Autodesk Inventor part; units mm, degrees
(part 6 of 18)
  line L1143 (-10073.7191, -10027.8364) -> (-10073.719, -10027.8366)
  line L1144 (-10073.9178, -10027.8132) -> (-10073.9177, -10027.8133)
  line L1145 (-10073.9467, -10028.0617) -> (-10073.9468, -10028.0615)
  line L1146 (-10073.7727, -10026.5717) -> (-10073.7726, -10026.5718)
  line L1147 (-10073.6031, -10026.8432) -> (-10073.8017, -10026.82)
  line L1148 (-10073.8017, -10026.82) -> (-10073.7727, -10026.5717)
  line L1149 (-10073.603, -10026.8433) -> (-10073.6031, -10026.8432)
  line L1150 (-10075.4902, -10026.6227) -> (-10074.0004, -10026.7968)
  line L1151 (-10074.0004, -10026.7968) -> (-10074.1164, -10027.79)
  line L1152 (-10074.1164, -10027.79) -> (-10075.6063, -10027.6159)
  line L1153 (-10075.6063, -10027.6159) -> (-10075.4902, -10026.6227)
  line L1154 (-10074.1959, -10026.9515) -> (-10075.3355, -10026.8184)
  line L1155 (-10074.0004, -10026.7968) -> (-10074.1959, -10026.9515)
  line L1156 (-10075.4902, -10026.6227) -> (-10075.3355, -10026.8184)
  line L1157 (-10075.3355, -10026.8184) -> (-10075.4106, -10027.4614)
  line L1158 (-10075.6063, -10027.6159) -> (-10075.4106, -10027.4614)
  line L1159 (-10075.4106, -10027.4614) -> (-10074.271, -10027.5945)
  line L1160 (-10074.1164, -10027.79) -> (-10074.271, -10027.5945)
  line L1161 (-10074.271, -10027.5945) -> (-10074.1959, -10026.9515)
  circle A25 centre (-10075.0634, -10027.176) radius 0.1
  line L1162 (-10074.92, -10027.3438) -> (-10075.2416, -10027.3062)
  line L1163 (-10075.2416, -10027.3062) -> (-10075.2416, -10027.3062)
  line L1164 (-10074.92, -10027.3438) -> (-10075.2416, -10027.3062)
  line L1165 (-10074.92, -10027.3438) -> (-10074.92, -10027.3438)
  line L1166 (-10075.2416, -10027.3062) -> (-10075.2068, -10027.0083)
  line L1167 (-10075.2068, -10027.0083) -> (-10074.8852, -10027.0458)
  line L1168 (-10074.8852, -10027.0459) -> (-10074.8852, -10027.0458)
  line L1169 (-10074.8852, -10027.0458) -> (-10074.92, -10027.3438)
  line L1170 (-10074.8852, -10027.0459) -> (-10074.92, -10027.3438)
  line L1171 (-10065.1619, -10026.3344) -> (-10065.1851, -10026.5331)
  line L1172 (-10065.162, -10026.3343) -> (-10065.1619, -10026.3344)
  line L1173 (-10065.1852, -10026.5329) -> (-10065.162, -10026.3343)
  line L1174 (-10065.1851, -10026.5331) -> (-10065.1852, -10026.5329)
  line L1175 (-10064.9136, -10026.3635) -> (-10065.1619, -10026.3344)
  line L1176 (-10064.9137, -10026.3633) -> (-10064.9136, -10026.3635)
  line L1177 (-10065.162, -10026.3343) -> (-10064.9137, -10026.3633)
  line L1178 (-10066.1552, -10026.2184) -> (-10066.3836, -10026.1917)
  line L1179 (-10066.1784, -10026.4169) -> (-10066.1784, -10026.417)
  line L1180 (-10066.1552, -10026.2183) -> (-10066.1784, -10026.4169)
  line L1181 (-10066.4035, -10026.1892) -> (-10066.1552, -10026.2183)
  line L1182 (-10066.4035, -10026.1894) -> (-10066.4035, -10026.1892)
  line L1183 (-10065.1851, -10026.5331) -> (-10066.1784, -10026.417)
  line L1184 (-10064.6931, -10024.4763) -> (-10064.9136, -10026.3635)
  line L1185 (-10065.1852, -10026.5329) -> (-10066.1784, -10026.4169)
  line L1186 (-10066.4035, -10026.1892) -> (-10066.183, -10024.3021)
  line L1187 (-10064.6932, -10024.4761) -> (-10064.9137, -10026.3633)
  line L1188 (-10065.9115, -10024.1324) -> (-10064.9183, -10024.2485)
  line L1189 (-10064.9182, -10024.2486) -> (-10064.9414, -10024.4471)
  line L1190 (-10064.6932, -10024.4761) -> (-10064.9415, -10024.4471)
  line L1191 (-10064.9415, -10024.4471) -> (-10064.9183, -10024.2485)
  line L1192 (-10064.9183, -10024.2485) -> (-10064.9182, -10024.2486)
  line L1193 (-10064.6931, -10024.4763) -> (-10064.6932, -10024.4761)
  line L1194 (-10065.9115, -10024.1324) -> (-10065.9347, -10024.3311)
  line L1195 (-10065.9347, -10024.3311) -> (-10066.183, -10024.3021)
  line L1196 (-10066.132, -10026.0196) -> (-10065.9579, -10024.5297)
  line L1197 (-10065.9579, -10024.5297) -> (-10064.9647, -10024.6458)
  line L1198 (-10064.9647, -10024.6458) -> (-10065.1388, -10026.1357)
  line L1199 (-10065.1388, -10026.1357) -> (-10066.132, -10026.0196)
  line L1200 (-10065.8032, -10024.7254) -> (-10065.9364, -10025.865)
  line L1201 (-10065.9579, -10024.5297) -> (-10065.8032, -10024.7254)
  line L1202 (-10066.132, -10026.0196) -> (-10065.9364, -10025.865)
  line L1203 (-10065.9364, -10025.865) -> (-10065.2934, -10025.9402)
  line L1204 (-10065.1388, -10026.1357) -> (-10065.2934, -10025.9402)
  line L1205 (-10065.2934, -10025.9402) -> (-10065.1602, -10024.8006)
  line L1206 (-10064.9647, -10024.6458) -> (-10065.1602, -10024.8006)
  line L1207 (-10065.1602, -10024.8006) -> (-10065.8032, -10024.7254)
  circle A26 centre (-10065.5787, -10025.5929) radius 0.1
  line L1208 (-10065.4109, -10025.4495) -> (-10065.4485, -10025.7711)
  line L1209 (-10065.4485, -10025.7712) -> (-10065.4485, -10025.7711)
  line L1210 (-10065.4109, -10025.4495) -> (-10065.4485, -10025.7712)
  line L1211 (-10065.4109, -10025.4495) -> (-10065.4109, -10025.4495)
  line L1212 (-10065.4485, -10025.7711) -> (-10065.7465, -10025.7363)
  line L1213 (-10065.7465, -10025.7363) -> (-10065.7465, -10025.7363)
  line L1214 (-10065.4485, -10025.7712) -> (-10065.7465, -10025.7363)
  line L1215 (-10065.7465, -10025.7363) -> (-10065.7089, -10025.4147)
  line L1216 (-10065.7089, -10025.4147) -> (-10065.4109, -10025.4495)
  line L1217 (-10077.2652, -10022.532) -> (-10077.0665, -10022.532)
  line L1218 (-10077.0665, -10022.532) -> (-10077.0665, -10022.782)
  line L1219 (-10077.0665, -10021.532) -> (-10077.2652, -10021.532)
  line L1220 (-10077.0665, -10021.282) -> (-10077.0665, -10021.532)
  line L1221 (-10075.017, -10021.282) -> (-10075.017, -10021.532)
  line L1222 (-10075.1793, -10021.282) -> (-10075.017, -10021.282)
  line L1223 (-10074.9807, -10021.532) -> (-10075.1793, -10021.532)
  line L1224 (-10075.1793, -10021.532) -> (-10075.1793, -10021.282)
  line L1225 (-10074.8184, -10021.532) -> (-10074.9807, -10021.532)
  line L1226 (-10074.8184, -10021.532) -> (-10074.8184, -10022.532)
  line L1227 (-10077.2652, -10022.532) -> (-10077.2652, -10021.532)
  line L1228 (-10077.0665, -10021.282) -> (-10075.1793, -10021.282)
  line L1229 (-10075.1793, -10022.782) -> (-10077.0665, -10022.782)
  line L1230 (-10074.9807, -10021.532) -> (-10074.9807, -10022.532)
  line L1231 (-10075.017, -10022.532) -> (-10075.017, -10022.782)
  line L1232 (-10075.1793, -10022.782) -> (-10075.1793, -10022.532)
  line L1233 (-10075.1793, -10022.532) -> (-10074.9807, -10022.532)
  line L1234 (-10074.9807, -10022.532) -> (-10074.8184, -10022.532)
  line L1235 (-10075.017, -10022.782) -> (-10075.1793, -10022.782)
  line L1236 (-10076.8679, -10021.532) -> (-10075.378, -10021.532)
  line L1237 (-10075.378, -10021.532) -> (-10075.378, -10022.532)
  line L1238 (-10075.378, -10022.532) -> (-10076.8679, -10022.532)
  line L1239 (-10076.8679, -10022.532) -> (-10076.8679, -10021.532)
  line L1240 (-10075.4372, -10021.7083) -> (-10076.5768, -10021.7083)
  line L1241 (-10075.378, -10021.532) -> (-10075.4372, -10021.7083)
  line L1242 (-10076.8679, -10021.532) -> (-10076.5768, -10021.7083)
  line L1243 (-10076.5768, -10021.7083) -> (-10076.5768, -10022.3557)
  line L1244 (-10076.8679, -10022.532) -> (-10076.5768, -10022.3557)
  line L1245 (-10076.5768, -10022.3557) -> (-10075.4372, -10022.3557)
  line L1246 (-10075.378, -10022.532) -> (-10075.4372, -10022.3557)
  line L1247 (-10075.4372, -10022.3557) -> (-10075.4372, -10021.7083)
  ellipse E653 centre (-10076.2961, -10022.032) end of major axis (-10076.2961, -10021.932) minor radius 0.0993
  ellipse E654 centre (-10076.2903, -10022.032) end of major axis (-10076.2903, -10021.932) minor radius 0.0993 (-10076.2903, -10022.132) -> (-10076.2903, -10021.932) ccw
  line L1248 (-10076.2903, -10022.132) -> (-10076.2961, -10022.132)
  line L1249 (-10076.2903, -10021.932) -> (-10076.2961, -10021.932)
  line L1250 (-10076.1295, -10022.182) -> (-10076.4512, -10022.182)
  line L1251 (-10076.1063, -10022.182) -> (-10076.1295, -10022.182)
  line L1252 (-10076.4512, -10022.182) -> (-10076.4512, -10021.882)
  line L1253 (-10076.4512, -10021.882) -> (-10076.1295, -10021.882)
  line L1254 (-10076.1063, -10021.882) -> (-10076.1295, -10021.882)
  line L1255 (-10076.1295, -10021.882) -> (-10076.1295, -10022.182)
  line L1256 (-10076.1063, -10021.882) -> (-10076.1063, -10022.182)
  line L1257 (-10066.5495, -10020.047) -> (-10066.5495, -10020.247)
  line L1258 (-10066.7118, -10020.247) -> (-10066.7118, -10020.047)
  line L1259 (-10066.5495, -10020.247) -> (-10066.7118, -10020.247)
  line L1260 (-10066.4635, -10020.047) -> (-10066.3012, -10020.047)
  line L1261 (-10066.7118, -10020.047) -> (-10066.4635, -10020.047)
  line L1262 (-10067.7051, -10020.047) -> (-10067.7051, -10020.247)
  line L1263 (-10067.9534, -10020.047) -> (-10067.7051, -10020.047)
  line L1264 (-10066.5495, -10017.947) -> (-10066.5495, -10018.147)
  line L1265 (-10066.4635, -10018.147) -> (-10066.7118, -10018.147)
  line L1266 (-10066.7118, -10018.147) -> (-10066.7118, -10017.947)
  line L1267 (-10066.7118, -10017.947) -> (-10066.5495, -10017.947)
  line L1268 (-10066.3012, -10018.147) -> (-10066.4635, -10018.147)
  line L1269 (-10066.3012, -10018.147) -> (-10066.3012, -10020.047)
  line L1270 (-10066.7118, -10020.247) -> (-10067.7051, -10020.247)
  line L1271 (-10067.9534, -10020.047) -> (-10067.9534, -10018.147)
  line L1272 (-10066.4635, -10018.147) -> (-10066.4635, -10020.047)
  line L1273 (-10067.7051, -10017.947) -> (-10066.7118, -10017.947)
  line L1274 (-10067.7051, -10017.947) -> (-10067.7051, -10018.147)
  line L1275 (-10067.7051, -10018.147) -> (-10067.9534, -10018.147)
  line L1276 (-10067.7051, -10019.847) -> (-10067.7051, -10018.347)
  line L1277 (-10067.7051, -10018.347) -> (-10066.7118, -10018.347)
  line L1278 (-10066.7118, -10018.347) -> (-10066.7118, -10019.847)
  line L1279 (-10066.7118, -10019.847) -> (-10067.7051, -10019.847)
  line L1280 (-10067.414, -10018.5233) -> (-10067.414, -10019.6707)
  line L1281 (-10067.7051, -10018.347) -> (-10067.414, -10018.5233)
  line L1282 (-10067.7051, -10019.847) -> (-10067.414, -10019.6707)
  line L1283 (-10067.414, -10019.6707) -> (-10066.771, -10019.6707)
  line L1284 (-10066.7118, -10019.847) -> (-10066.771, -10019.6707)
  line L1285 (-10066.771, -10019.6707) -> (-10066.771, -10018.5233)
  line L1286 (-10066.7118, -10018.347) -> (-10066.771, -10018.5233)
  line L1287 (-10066.771, -10018.5233) -> (-10067.414, -10018.5233)
  ellipse E655 centre (-10067.1215, -10019.3589) end of major axis (-10067.1215, -10019.2589) minor radius 0.0993
  ellipse E656 centre (-10067.1157, -10019.3589) end of major axis (-10067.1157, -10019.2589) minor radius 0.0993 (-10067.1157, -10019.4589) -> (-10067.1157, -10019.2589) ccw
  line L1288 (-10067.1157, -10019.4589) -> (-10067.1215, -10019.4589)
  line L1289 (-10067.1157, -10019.2589) -> (-10067.1215, -10019.2589)
  line L1290 (-10066.9667, -10019.197) -> (-10066.9667, -10019.5208)
  line L1291 (-10066.9435, -10019.5208) -> (-10066.9667, -10019.5208)
  line L1292 (-10066.9435, -10019.197) -> (-10066.9435, -10019.5208)
  line L1293 (-10066.9435, -10019.197) -> (-10066.9667, -10019.197)
  line L1294 (-10066.9667, -10019.5208) -> (-10067.2647, -10019.5208)
  line L1295 (-10067.2647, -10019.5208) -> (-10067.2647, -10019.197)
  line L1296 (-10067.2647, -10019.197) -> (-10066.9667, -10019.197)
  line L1297 (-10064.9414, -10013.7468) -> (-10064.9182, -10013.9454)
  line L1298 (-10064.9183, -10013.9455) -> (-10064.9415, -10013.7468)
  line L1299 (-10064.9182, -10013.9454) -> (-10064.9183, -10013.9455)
  line L1300 (-10064.6932, -10013.7178) -> (-10064.6931, -10013.7177)
  line L1301 (-10064.9415, -10013.7468) -> (-10064.6932, -10013.7178)
  line L1302 (-10065.9347, -10013.8629) -> (-10065.9115, -10014.0615)
  line L1303 (-10066.183, -10013.8919) -> (-10065.9347, -10013.8629)
  line L1304 (-10066.3836, -10012.0023) -> (-10066.1552, -10011.9756)
  line L1305 (-10066.4035, -10012.0047) -> (-10066.4035, -10012.0046)
  line L1306 (-10066.1784, -10011.7771) -> (-10066.1552, -10011.9757)
  line L1307 (-10066.1552, -10011.9757) -> (-10066.4035, -10012.0047)
  line L1308 (-10066.1784, -10011.7769) -> (-10066.1784, -10011.7771)
  line L1309 (-10066.1784, -10011.7769) -> (-10065.1851, -10011.6609)
  line L1310 (-10064.9136, -10011.8305) -> (-10064.6931, -10013.7177)
  line L1311 (-10064.9183, -10013.9455) -> (-10065.9115, -10014.0615)
  line L1312 (-10066.183, -10013.8919) -> (-10066.4035, -10012.0047)
  line L1313 (-10064.9137, -10011.8307) -> (-10064.6932, -10013.7178)
  line L1314 (-10066.1784, -10011.7771) -> (-10065.1852, -10011.661)
  line L1315 (-10065.1851, -10011.6609) -> (-10065.1619, -10011.8595)
  line L1316 (-10065.1619, -10011.8595) -> (-10064.9136, -10011.8305)
  line L1317 (-10064.9137, -10011.8307) -> (-10065.162, -10011.8597)
  line L1318 (-10065.162, -10011.8597) -> (-10065.1852, -10011.661)
  line L1319 (-10065.1852, -10011.661) -> (-10065.1851, -10011.6609)
  line L1320 (-10065.162, -10011.8597) -> (-10065.1619, -10011.8595)
  line L1321 (-10064.9136, -10011.8305) -> (-10064.9137, -10011.8307)
  line L1322 (-10065.9579, -10013.6642) -> (-10066.132, -10012.1744)
  line L1323 (-10066.132, -10012.1744) -> (-10065.1388, -10012.0583)
  line L1324 (-10065.1388, -10012.0583) -> (-10064.9647, -10013.5482)
  line L1325 (-10064.9647, -10013.5482) -> (-10065.9579, -10013.6642)
  line L1326 (-10065.9364, -10012.329) -> (-10065.8032, -10013.4685)
  line L1327 (-10066.132, -10012.1744) -> (-10065.9364, -10012.329)
  line L1328 (-10065.9579, -10013.6642) -> (-10065.8032, -10013.4685)
  line L1329 (-10065.8032, -10013.4685) -> (-10065.1602, -10013.3934)
  line L1330 (-10064.9647, -10013.5482) -> (-10065.1602, -10013.3934)
  line L1331 (-10065.1602, -10013.3934) -> (-10065.2934, -10012.2538)
  line L1332 (-10065.1388, -10012.0583) -> (-10065.2934, -10012.2538)
  line L1333 (-10065.2934, -10012.2538) -> (-10065.9364, -10012.329)
  circle A27 centre (-10065.5179, -10013.1214) radius 0.1
  line L1334 (-10065.3877, -10012.9431) -> (-10065.3501, -10013.2648)
  line L1335 (-10065.3501, -10013.2647) -> (-10065.3501, -10013.2648)
  line L1336 (-10065.3877, -10012.9431) -> (-10065.3501, -10013.2647)
  line L1337 (-10065.3877, -10012.9431) -> (-10065.3877, -10012.9431)
  line L1338 (-10065.3501, -10013.2648) -> (-10065.6481, -10013.2996)
  line L1339 (-10065.6481, -10013.2996) -> (-10065.6857, -10012.9779)
  line L1340 (-10065.6857, -10012.9779) -> (-10065.6857, -10012.9779)
  line L1341 (-10065.6857, -10012.9779) -> (-10065.3877, -10012.9431)
  line L1342 (-10065.6857, -10012.9779) -> (-10065.3877, -10012.9431)
  line L1343 (-10079.6036, -10026.2937) -> (-10079.8027, -10026.2748)
  line L1344 (-10079.8027, -10026.2747) -> (-10079.6036, -10026.2936)
  line L1345 (-10079.8027, -10026.2748) -> (-10079.8027, -10026.2747)
  line L1346 (-10079.6272, -10026.5425) -> (-10079.6272, -10026.5426)
  line L1347 (-10079.6036, -10026.2936) -> (-10079.6272, -10026.5425)
  line L1348 (-10079.5092, -10025.298) -> (-10079.7083, -10025.2792)
  line L1349 (-10079.4856, -10025.0492) -> (-10079.5092, -10025.298)
  line L1350 (-10079.407, -10026.5634) -> (-10079.6272, -10026.5426)
  line L1351 (-10079.8027, -10026.2747) -> (-10079.7083, -10025.2792)
  line L1352 (-10079.4856, -10025.0492) -> (-10077.5941, -10025.2284)
  line L1353 (-10077.8748, -10026.7086) -> (-10079.6272, -10026.5425)
  line L1354 (-10077.4186, -10025.4962) -> (-10077.433, -10025.6486)
  line L1355 (-10077.5941, -10025.2284) -> (-10077.5941, -10025.2285)
  line L1356 (-10077.4186, -10025.4962) -> (-10077.6177, -10025.4773)
  line L1357 (-10077.6177, -10025.4773) -> (-10077.5941, -10025.2284)
  line L1358 (-10077.4186, -10025.4963) -> (-10077.4186, -10025.4962)
  line L1359 (-10079.3101, -10025.3169) -> (-10077.8168, -10025.4585)
  line L1360 (-10077.8168, -10025.4585) -> (-10077.9112, -10026.454)
  line L1361 (-10077.9112, -10026.454) -> (-10079.4045, -10026.3125)
  line L1362 (-10079.4045, -10026.3125) -> (-10079.3101, -10025.3169)
  line L1363 (-10078.009, -10025.6174) -> (-10079.1512, -10025.5092)
  line L1364 (-10077.8168, -10025.4585) -> (-10078.009, -10025.6174)
  line L1365 (-10079.3101, -10025.3169) -> (-10079.1512, -10025.5092)
  line L1366 (-10079.1512, -10025.5092) -> (-10079.2123, -10026.1536)
  line L1367 (-10079.4045, -10026.3125) -> (-10079.2123, -10026.1536)
  line L1368 (-10079.2123, -10026.1536) -> (-10078.0701, -10026.2619)
  line L1369 (-10077.9112, -10026.454) -> (-10078.0701, -10026.2619)
  line L1370 (-10078.0701, -10026.2619) -> (-10078.009, -10025.6174)
  circle A28 centre (-10078.8714, -10025.8608) radius 0.1
  line L1371 (-10078.7243, -10026.0254) -> (-10079.0467, -10025.9949)
  line L1372 (-10078.7243, -10026.0254) -> (-10079.0467, -10025.9949)
  line L1373 (-10079.0467, -10025.9949) -> (-10079.0184, -10025.6962)
  line L1374 (-10079.0184, -10025.6962) -> (-10078.696, -10025.7267)
  line L1375 (-10078.696, -10025.7267) -> (-10078.7243, -10026.0254)
  line L1376 (-10068.9906, -10024.8034) -> (-10068.9906, -10024.8035)
  line L1377 (-10069.0095, -10025.0025) -> (-10068.9906, -10024.8034)
  line L1378 (-10069.0095, -10025.0026) -> (-10069.0095, -10025.0025)
  line L1379 (-10068.7417, -10024.827) -> (-10068.7417, -10024.8271)
  line L1380 (-10068.9906, -10024.8034) -> (-10068.7417, -10024.827)
  line L1381 (-10070.005, -10024.9081) -> (-10070.005, -10024.9082)
  line L1382 (-10069.9861, -10024.709) -> (-10070.005, -10024.9081)
  line L1383 (-10070.235, -10024.6854) -> (-10069.9861, -10024.709)
  line L1384 (-10070.235, -10024.6856) -> (-10070.235, -10024.6854)
  line L1385 (-10069.0095, -10025.0025) -> (-10070.005, -10024.9081)
  line L1386 (-10070.235, -10024.6854) -> (-10070.0557, -10022.7939)
  line L1387 (-10068.5624, -10022.9355) -> (-10068.7417, -10024.827)
  line L1388 (-10069.788, -10022.6184) -> (-10068.7924, -10022.7128)
  line L1389 (-10068.5624, -10022.9355) -> (-10068.8113, -10022.9119)
  line L1390 (-10068.8113, -10022.9119) -> (-10068.7924, -10022.7128)
  line L1391 (-10068.7924, -10022.7128) -> (-10068.7924, -10022.7129)
  line L1392 (-10068.5624, -10022.9356) -> (-10068.5624, -10022.9355)
  line L1393 (-10069.788, -10022.6184) -> (-10069.8069, -10022.8175)
  line L1394 (-10069.8069, -10022.8175) -> (-10070.0557, -10022.7939)
  line L1395 (-10069.9673, -10024.5099) -> (-10069.8257, -10023.0166)
  line L1396 (-10069.8257, -10023.0166) -> (-10068.8302, -10023.111)
  line L1397 (-10068.8302, -10023.111) -> (-10068.9717, -10024.6043)
  line L1398 (-10068.9717, -10024.6043) -> (-10069.9673, -10024.5099)
  line L1399 (-10069.6668, -10023.2089) -> (-10069.7751, -10024.3511)
  line L1400 (-10069.8257, -10023.0166) -> (-10069.6668, -10023.2089)
  line L1401 (-10069.9673, -10024.5099) -> (-10069.7751, -10024.3511)
  line L1402 (-10069.7751, -10024.3511) -> (-10069.1306, -10024.4122)
  line L1403 (-10068.9717, -10024.6043) -> (-10069.1306, -10024.4122)
  line L1404 (-10069.1306, -10024.4122) -> (-10069.0224, -10023.27)
  line L1405 (-10068.8302, -10023.111) -> (-10069.0224, -10023.27)
  line L1406 (-10069.0224, -10023.27) -> (-10069.6668, -10023.2089)
  circle A29 centre (-10069.4234, -10024.0713) radius 0.1
  line L1407 (-10069.2588, -10023.9242) -> (-10069.2894, -10024.2466)
  line L1408 (-10069.2894, -10024.2466) -> (-10069.5881, -10024.2183)
  line L1409 (-10069.2894, -10024.2466) -> (-10069.5881, -10024.2183)
  line L1410 (-10069.5881, -10024.2183) -> (-10069.5575, -10023.8959)
  line L1411 (-10069.5575, -10023.8959) -> (-10069.2588, -10023.9242)
  line L1412 (-10080.8297, -10022.532) -> (-10080.6306, -10022.532)
  line L1413 (-10080.6306, -10022.532) -> (-10080.6306, -10022.782)
  line L1414 (-10080.6306, -10021.532) -> (-10080.8297, -10021.532)
  line L1415 (-10080.6306, -10021.282) -> (-10080.6306, -10021.532)
  line L1416 (-10080.8297, -10022.532) -> (-10080.8297, -10021.532)
  line L1417 (-10080.6306, -10021.282) -> (-10078.8245, -10021.282)
  line L1418 (-10078.8245, -10022.782) -> (-10080.6306, -10022.782)
  line L1419 (-10080.4314, -10021.532) -> (-10079.0234, -10021.532)
  line L1420 (-10079.0234, -10022.532) -> (-10080.4314, -10022.532)
  line L1421 (-10080.4314, -10022.532) -> (-10080.4314, -10021.532)
  line L1422 (-10079.6809, -10021.7083) -> (-10080.1616, -10021.7083)
  line L1423 (-10080.4314, -10021.532) -> (-10080.1616, -10021.7083)
  line L1424 (-10080.1616, -10021.7083) -> (-10080.1616, -10022.3557)
  line L1425 (-10080.4314, -10022.532) -> (-10080.1616, -10022.3557)
  line L1426 (-10080.1616, -10022.3557) -> (-10079.6809, -10022.3557)
  ellipse E657 centre (-10079.8748, -10022.032) end of major axis (-10079.8748, -10021.932) minor radius 0.0996
  ellipse E658 centre (-10079.8701, -10022.032) end of major axis (-10079.8701, -10021.932) minor radius 0.0996 (-10079.8701, -10022.132) -> (-10079.8701, -10021.932) ccw
  line L1427 (-10079.8701, -10022.132) -> (-10079.8748, -10022.132)
  line L1428 (-10079.8701, -10021.932) -> (-10079.8748, -10021.932)
  line L1429 (-10079.7089, -10022.182) -> (-10080.0313, -10022.182)
  line L1430 (-10079.69, -10022.182) -> (-10079.7089, -10022.182)
  line L1431 (-10080.0313, -10022.182) -> (-10080.0313, -10021.882)
  line L1432 (-10080.0313, -10021.882) -> (-10079.7089, -10021.882)
  line L1433 (-10079.69, -10021.882) -> (-10079.7089, -10021.882)
  line L1434 (-10079.7089, -10021.882) -> (-10079.7089, -10022.182)
  line L1435 (-10079.69, -10021.882) -> (-10079.69, -10022.182)
  line L1436 (-10070.252, -10020.247) -> (-10070.252, -10020.047)
  line L1437 (-10070.2216, -10020.247) -> (-10070.252, -10020.247)
  line L1438 (-10070.0031, -10020.047) -> (-10069.9732, -10020.047)
  line L1439 (-10070.252, -10020.047) -> (-10070.0031, -10020.047)
  line L1440 (-10071.2476, -10020.047) -> (-10071.2476, -10020.247)
  line L1441 (-10071.4965, -10020.047) -> (-10071.2476, -10020.047)
  line L1442 (-10070.252, -10020.247) -> (-10071.2476, -10020.247)
  line L1443 (-10071.4965, -10020.047) -> (-10071.4965, -10018.147)
  line L1444 (-10070.0031, -10018.147) -> (-10070.0031, -10020.047)
  line L1445 (-10071.2476, -10017.947) -> (-10070.252, -10017.947)
  line L1446 (-10070.0031, -10018.147) -> (-10070.252, -10018.147)
  line L1447 (-10070.252, -10018.147) -> (-10070.252, -10017.947)
  line L1448 (-10070.252, -10017.947) -> (-10070.2216, -10017.947)
  line L1449 (-10069.9732, -10018.147) -> (-10070.0031, -10018.147)
  line L1450 (-10071.2476, -10017.947) -> (-10071.2476, -10018.147)
  line L1451 (-10071.2476, -10018.147) -> (-10071.4965, -10018.147)
  line L1452 (-10071.2476, -10019.847) -> (-10071.2476, -10018.347)
  line L1453 (-10071.2476, -10018.347) -> (-10070.252, -10018.347)
  line L1454 (-10070.252, -10018.347) -> (-10070.252, -10019.847)
  line L1455 (-10070.252, -10019.847) -> (-10071.2476, -10019.847)
  line L1456 (-10071.2476, -10018.347) -> (-10071.1549, -10018.4076)
  line L1457 (-10071.2476, -10019.847) -> (-10071.1549, -10019.7864)
  line L1458 (-10070.252, -10019.847) -> (-10070.2784, -10019.7898)
  line L1459 (-10070.252, -10018.347) -> (-10070.2784, -10018.4042)
  line L1460 (-10068.7924, -10015.4812) -> (-10068.8113, -10015.2821)
  line L1461 (-10068.7924, -10015.4811) -> (-10068.7924, -10015.4812)
  line L1462 (-10068.5624, -10015.2585) -> (-10068.5624, -10015.2584)
  line L1463 (-10068.8113, -10015.2821) -> (-10068.5624, -10015.2585)
  line L1464 (-10069.8069, -10015.3765) -> (-10069.788, -10015.5756)
  line L1465 (-10070.0557, -10015.4001) -> (-10069.8069, -10015.3765)
  line L1466 (-10068.7924, -10015.4812) -> (-10069.788, -10015.5756)
  line L1467 (-10070.0557, -10015.4001) -> (-10070.235, -10013.5085)
  line L1468 (-10068.7417, -10013.367) -> (-10068.5624, -10015.2585)
  line L1469 (-10070.005, -10013.2858) -> (-10069.0095, -10013.1915)
  line L1470 (-10070.235, -10013.5085) -> (-10070.235, -10013.5084)
  line L1471 (-10070.005, -10013.2858) -> (-10069.9861, -10013.4849)
  line L1472 (-10069.9861, -10013.4849) -> (-10070.235, -10013.5085)
  line L1473 (-10070.005, -10013.2857) -> (-10070.005, -10013.2858)
  line L1474 (-10068.7417, -10013.367) -> (-10068.9906, -10013.3906)
  line L1475 (-10068.9906, -10013.3906) -> (-10069.0095, -10013.1915)
  line L1476 (-10069.0095, -10013.1915) -> (-10069.0095, -10013.1914)
  line L1477 (-10068.9906, -10013.3906) -> (-10068.9906, -10013.3905)
  line L1478 (-10068.7417, -10013.3669) -> (-10068.7417, -10013.367)
  line L1479 (-10069.8257, -10015.1774) -> (-10069.9673, -10013.684)
  line L1480 (-10069.9673, -10013.684) -> (-10068.9717, -10013.5897)
  line L1481 (-10068.9717, -10013.5897) -> (-10068.8302, -10015.083)
  line L1482 (-10068.8302, -10015.083) -> (-10069.8257, -10015.1774)
  line L1483 (-10069.7751, -10013.8429) -> (-10069.6668, -10014.9851)
  line L1484 (-10069.9673, -10013.684) -> (-10069.7751, -10013.8429)
  line L1485 (-10069.8257, -10015.1774) -> (-10069.6668, -10014.9851)
  line L1486 (-10069.6668, -10014.9851) -> (-10069.0224, -10014.924)
  line L1487 (-10068.8302, -10015.083) -> (-10069.0224, -10014.924)
  line L1488 (-10069.0224, -10014.924) -> (-10069.1306, -10013.7818)
  line L1489 (-10068.9717, -10013.5897) -> (-10069.1306, -10013.7818)
  line L1490 (-10069.1306, -10013.7818) -> (-10069.7751, -10013.8429)
  circle A30 centre (-10069.374, -10014.6442) radius 0.1
  line L1491 (-10069.24, -10014.4689) -> (-10069.2094, -10014.7912)
  line L1492 (-10069.2094, -10014.7912) -> (-10069.5081, -10014.8195)
  line L1493 (-10069.5081, -10014.8195) -> (-10069.5386, -10014.4972)
  line L1494 (-10069.5386, -10014.4972) -> (-10069.24, -10014.4689)
  line L1495 (-10069.5386, -10014.4972) -> (-10069.24, -10014.4688)
  line L1496 (-10051.002, -10021.597) -> (-10051.202, -10021.597)
  line L1497 (-10051.202, -10021.597) -> (-10051.202, -10021.347)
  line L1498 (-10051.202, -10022.597) -> (-10051.002, -10022.597)
  line L1499 (-10051.202, -10022.847) -> (-10051.202, -10022.597)
  line L1500 (-10051.002, -10021.597) -> (-10051.002, -10022.597)
  line L1501 (-10051.202, -10022.847) -> (-10053.102, -10022.847)
  line L1502 (-10053.102, -10021.347) -> (-10051.202, -10021.347)
  line L1503 (-10053.302, -10022.597) -> (-10053.302, -10021.597)
  line L1504 (-10053.102, -10021.347) -> (-10053.102, -10021.597)
  line L1505 (-10053.102, -10021.597) -> (-10053.302, -10021.597)
  line L1506 (-10053.302, -10022.597) -> (-10053.102, -10022.597)
  line L1507 (-10053.102, -10022.597) -> (-10053.102, -10022.847)
  line L1508 (-10051.402, -10022.597) -> (-10052.902, -10022.597)
  line L1509 (-10052.902, -10022.597) -> (-10052.902, -10021.597)
  line L1510 (-10052.902, -10021.597) -> (-10051.402, -10021.597)
  line L1511 (-10051.402, -10021.597) -> (-10051.402, -10022.597)
  line L1512 (-10052.7257, -10022.4207) -> (-10051.5783, -10022.4207)
  line L1513 (-10052.902, -10022.597) -> (-10052.7257, -10022.4207)
  line L1514 (-10051.402, -10022.597) -> (-10051.5783, -10022.4207)
  line L1515 (-10051.5783, -10022.4207) -> (-10051.5783, -10021.7733)
  line L1516 (-10051.402, -10021.597) -> (-10051.5783, -10021.7733)
  line L1517 (-10051.5783, -10021.7733) -> (-10052.7257, -10021.7733)
  line L1518 (-10052.902, -10021.597) -> (-10052.7257, -10021.7733)
  line L1519 (-10052.7257, -10021.7733) -> (-10052.7257, -10022.4207)
  circle A31 centre (-10051.8901, -10022.097) radius 0.1
  line L1520 (-10052.052, -10021.947) -> (-10051.7282, -10021.947)
  line L1521 (-10051.7282, -10021.947) -> (-10051.7282, -10022.247)
  line L1522 (-10051.7282, -10022.247) -> (-10052.052, -10022.247)
  line L1523 (-10052.052, -10022.247) -> (-10052.052, -10021.947)
  line L1524 (-10061.6, -10017.947) -> (-10061.6, -10018.147)
  line L1525 (-10061.6, -10018.147) -> (-10061.85, -10018.147)
  line L1526 (-10060.6, -10018.147) -> (-10060.6, -10017.947)
  line L1527 (-10060.35, -10018.147) -> (-10060.6, -10018.147)
  line L1528 (-10061.6, -10017.947) -> (-10060.6, -10017.947)
  line L1529 (-10060.35, -10018.147) -> (-10060.35, -10020.047)
  line L1530 (-10061.85, -10020.047) -> (-10061.85, -10018.147)
  line L1531 (-10060.6, -10020.247) -> (-10061.6, -10020.247)
  line L1532 (-10061.85, -10020.047) -> (-10061.6, -10020.047)
  line L1533 (-10061.6, -10020.047) -> (-10061.6, -10020.247)
  line L1534 (-10060.6, -10020.247) -> (-10060.6, -10020.047)
  line L1535 (-10060.6, -10020.047) -> (-10060.35, -10020.047)
  line L1536 (-10060.6, -10018.347) -> (-10060.6, -10019.847)
  line L1537 (-10060.6, -10019.847) -> (-10061.6, -10019.847)
  line L1538 (-10061.6, -10019.847) -> (-10061.6, -10018.347)
  line L1539 (-10061.6, -10018.347) -> (-10060.6, -10018.347)
  line L1540 (-10060.7763, -10019.6707) -> (-10060.7763, -10018.5233)
  line L1541 (-10060.6, -10019.847) -> (-10060.7763, -10019.6707)
  line L1542 (-10060.6, -10018.347) -> (-10060.7763, -10018.5233)
  line L1543 (-10060.7763, -10018.5233) -> (-10061.4237, -10018.5233)
  line L1544 (-10061.6, -10018.347) -> (-10061.4237, -10018.5233)
  line L1545 (-10061.4237, -10018.5233) -> (-10061.4237, -10019.6707)
  line L1546 (-10061.6, -10019.847) -> (-10061.4237, -10019.6707)
  line L1547 (-10061.4237, -10019.6707) -> (-10060.7763, -10019.6707)
  circle A32 centre (-10061.1, -10018.8351) radius 0.1
  line L1548 (-10061.25, -10018.997) -> (-10061.25, -10018.6732)
  line L1549 (-10061.25, -10018.6732) -> (-10060.95, -10018.6732)
  line L1550 (-10060.95, -10018.6732) -> (-10060.95, -10018.997)
  line L1551 (-10060.95, -10018.997) -> (-10061.25, -10018.997)
  line L1552 (-10051.002, -10015.597) -> (-10051.202, -10015.597)
  line L1553 (-10051.202, -10015.597) -> (-10051.202, -10015.347)
  line L1554 (-10051.202, -10016.597) -> (-10051.002, -10016.597)
  line L1555 (-10051.202, -10016.847) -> (-10051.202, -10016.597)
  line L1556 (-10051.002, -10015.597) -> (-10051.002, -10016.597)
  line L1557 (-10051.202, -10016.847) -> (-10053.102, -10016.847)
  line L1558 (-10053.102, -10015.347) -> (-10051.202, -10015.347)
  line L1559 (-10053.302, -10016.597) -> (-10053.302, -10015.597)
  line L1560 (-10053.102, -10015.347) -> (-10053.102, -10015.597)
  line L1561 (-10053.102, -10015.597) -> (-10053.302, -10015.597)
  line L1562 (-10053.302, -10016.597) -> (-10053.102, -10016.597)
  line L1563 (-10053.102, -10016.597) -> (-10053.102, -10016.847)
  line L1564 (-10051.402, -10016.597) -> (-10052.902, -10016.597)
  line L1565 (-10052.902, -10016.597) -> (-10052.902, -10015.597)
  line L1566 (-10052.902, -10015.597) -> (-10051.402, -10015.597)
  line L1567 (-10051.402, -10015.597) -> (-10051.402, -10016.597)
  line L1568 (-10052.7257, -10016.4207) -> (-10051.5783, -10016.4207)
  line L1569 (-10052.902, -10016.597) -> (-10052.7257, -10016.4207)
  line L1570 (-10051.402, -10016.597) -> (-10051.5783, -10016.4207)
  line L1571 (-10051.5783, -10016.4207) -> (-10051.5783, -10015.7733)
  line L1572 (-10051.402, -10015.597) -> (-10051.5783, -10015.7733)
  line L1573 (-10051.5783, -10015.7733) -> (-10052.7257, -10015.7733)
  line L1574 (-10052.902, -10015.597) -> (-10052.7257, -10015.7733)
  line L1575 (-10052.7257, -10015.7733) -> (-10052.7257, -10016.4207)
  circle A33 centre (-10051.8901, -10016.097) radius 0.1
  line L1576 (-10052.052, -10015.947) -> (-10051.7282, -10015.947)
  line L1577 (-10051.7282, -10015.947) -> (-10051.7282, -10016.247)
  line L1578 (-10051.7282, -10016.247) -> (-10052.052, -10016.247)
  line L1579 (-10052.052, -10016.247) -> (-10052.052, -10015.947)
  line L1580 (-10079.0234, -10015.662) -> (-10078.8245, -10015.662)
  line L1581 (-10078.8245, -10015.662) -> (-10078.8245, -10015.412)
  line L1582 (-10078.8245, -10016.662) -> (-10079.0234, -10016.662)
  line L1583 (-10078.8245, -10016.912) -> (-10078.8245, -10016.662)
  line L1584 (-10079.0234, -10015.662) -> (-10079.0234, -10016.662)
  line L1585 (-10078.8245, -10016.912) -> (-10077.0665, -10016.912)
  line L1586 (-10077.0665, -10015.412) -> (-10078.8245, -10015.412)
  line L1587 (-10078.6256, -10016.662) -> (-10077.2652, -10016.662)
  line L1588 (-10078.6256, -10015.662) -> (-10078.6256, -10016.662)
  line L1589 (-10077.2652, -10015.662) -> (-10078.6256, -10015.662)
  line L1590 (-10078.6256, -10016.662) -> (-10078.3721, -10016.502)
  line L1591 (-10078.6256, -10015.662) -> (-10078.3721, -10015.822)
  ellipse E659 centre (-10078.0621, -10016.162) end of major axis (-10078.0621, -10016.262) minor radius 0.0995
  ellipse E660 centre (-10078.0569, -10016.162) end of major axis (-10078.0569, -10016.262) minor radius 0.0995 (-10078.0569, -10016.262) -> (-10078.0569, -10016.062) ccw
  line L1592 (-10078.0621, -10016.062) -> (-10078.0569, -10016.062)
  line L1593 (-10078.0621, -10016.262) -> (-10078.0569, -10016.262)
  line L1594 (-10077.8958, -10016.012) -> (-10078.2179, -10016.012)
  line L1595 (-10077.8853, -10016.012) -> (-10077.8958, -10016.012)
  line L1596 (-10078.2179, -10016.012) -> (-10078.2179, -10016.312)
  line L1597 (-10078.2179, -10016.312) -> (-10077.8958, -10016.312)
  line L1598 (-10077.8853, -10016.312) -> (-10077.8958, -10016.312)
  line L1599 (-10077.8958, -10016.312) -> (-10077.8958, -10016.012)
  line L1600 (-10077.6915, -10011.3153) -> (-10077.8903, -10011.3361)
  line L1601 (-10077.8903, -10011.3361) -> (-10077.8904, -10011.3364)
  line L1602 (-10077.8904, -10011.3364) -> (-10077.6915, -10011.3156)
  line L1603 (-10077.6915, -10011.3156) -> (-10077.7175, -10011.0669)
  line L1604 (-10077.7175, -10011.0669) -> (-10077.7174, -10011.0667)
  line L1605 (-10077.5874, -10012.3101) -> (-10077.7864, -10012.3309)
  line L1606 (-10077.5614, -10012.5588) -> (-10077.5874, -10012.3101)
  line L1607 (-10075.9732, -10010.8842) -> (-10077.7174, -10011.0667)
  line L1608 (-10075.4988, -10012.0914) -> (-10075.5264, -10011.8272)
  line L1609 (-10077.8904, -10011.3364) -> (-10077.7864, -10012.3309)
  line L1610 (-10077.5614, -10012.5588) -> (-10075.6718, -10012.3611)
  line L1611 (-10075.4989, -10012.0916) -> (-10075.6029, -10011.097)
  line L1612 (-10075.8278, -10010.8692) -> (-10077.7175, -10011.0669)
  line L1613 (-10075.6717, -10012.3608) -> (-10075.6977, -10012.1124)
  line L1614 (-10075.6718, -10012.3611) -> (-10075.6717, -10012.3608)
  line L1615 (-10075.6978, -10012.1124) -> (-10075.6718, -10012.3611)
  line L1616 (-10075.4989, -10012.0916) -> (-10075.6978, -10012.1124)
  line L1617 (-10075.4988, -10012.0914) -> (-10075.4989, -10012.0916)
  line L1618 (-10075.8018, -10011.1178) -> (-10075.6029, -10011.097)
  line L1619 (-10075.8278, -10010.8692) -> (-10075.8018, -10011.1178)
  line L1620 (-10077.3885, -10012.2893) -> (-10075.8967, -10012.1332)
  line L1621 (-10077.4926, -10011.2947) -> (-10077.3885, -10012.2893)
  line L1622 (-10076.0007, -10011.1387) -> (-10077.4926, -10011.2947)
  line L1623 (-10075.8967, -10012.1332) -> (-10076.0007, -10011.1387)
  line L1624 (-10076.0903, -10011.976) -> (-10077.2315, -10012.0954)
  line L1625 (-10077.3885, -10012.2893) -> (-10077.2315, -10012.0954)
  line L1626 (-10075.8967, -10012.1332) -> (-10076.0903, -10011.976)
  line L1627 (-10077.2315, -10012.0954) -> (-10077.2988, -10011.4516)
  line L1628 (-10077.4926, -10011.2947) -> (-10077.2988, -10011.4516)
  line L1629 (-10077.2988, -10011.4516) -> (-10076.1577, -10011.3322)
  line L1630 (-10076.0007, -10011.1387) -> (-10076.1577, -10011.3322)
  line L1631 (-10076.1577, -10011.3322) -> (-10076.0903, -10011.976)
  circle A34 centre (-10076.9551, -10011.7411) radius 0.1
  line L1632 (-10076.8097, -10011.5751) -> (-10077.1317, -10011.6088)
  line L1633 (-10076.8096, -10011.575) -> (-10076.8097, -10011.5751)
  line L1634 (-10076.8096, -10011.575) -> (-10077.1317, -10011.6087)
  line L1635 (-10077.1317, -10011.6087) -> (-10077.1317, -10011.6088)
  line L1636 (-10077.1317, -10011.6088) -> (-10077.1005, -10011.9071)
  line L1637 (-10077.1005, -10011.9071) -> (-10076.7784, -10011.8735)
  line L1638 (-10076.7784, -10011.8734) -> (-10076.7784, -10011.8735)
  line L1639 (-10076.7784, -10011.8735) -> (-10076.8097, -10011.5751)
  line L1640 (-10076.7784, -10011.8734) -> (-10076.8096, -10011.575)
  line L1641 (-10077.2652, -10015.662) -> (-10077.0665, -10015.662)
  line L1642 (-10077.0665, -10015.662) -> (-10077.0665, -10015.412)
  line L1643 (-10077.0665, -10016.662) -> (-10077.2652, -10016.662)
  line L1644 (-10077.0665, -10016.912) -> (-10077.0665, -10016.662)
  line L1645 (-10075.017, -10015.662) -> (-10075.017, -10015.412)
  line L1646 (-10075.1793, -10015.662) -> (-10074.9807, -10015.662)
  line L1647 (-10075.1793, -10015.412) -> (-10075.1793, -10015.662)
  line L1648 (-10074.9807, -10015.662) -> (-10074.8184, -10015.662)
  line L1649 (-10075.017, -10015.412) -> (-10075.1793, -10015.412)
  line L1650 (-10074.8184, -10016.662) -> (-10074.8184, -10015.662)
  line L1651 (-10077.2652, -10015.662) -> (-10077.2652, -10016.662)
  line L1652 (-10077.0665, -10016.912) -> (-10075.1793, -10016.912)
  line L1653 (-10074.9807, -10016.662) -> (-10074.9807, -10015.662)
  line L1654 (-10075.1793, -10015.412) -> (-10077.0665, -10015.412)
  line L1655 (-10075.017, -10016.912) -> (-10075.017, -10016.662)
  line L1656 (-10075.1793, -10016.912) -> (-10075.017, -10016.912)
  line L1657 (-10075.1793, -10016.662) -> (-10075.1793, -10016.912)
  line L1658 (-10074.9807, -10016.662) -> (-10075.1793, -10016.662)
  line L1659 (-10074.8184, -10016.662) -> (-10074.9807, -10016.662)
  line L1660 (-10076.8679, -10016.662) -> (-10075.378, -10016.662)
  line L1661 (-10076.8679, -10015.662) -> (-10076.8679, -10016.662)
  line L1662 (-10075.378, -10015.662) -> (-10076.8679, -10015.662)
  line L1663 (-10075.378, -10016.662) -> (-10075.378, -10015.662)
  line L1664 (-10075.4372, -10016.4857) -> (-10076.5768, -10016.4857)
  line L1665 (-10076.8679, -10016.662) -> (-10076.5768, -10016.4857)
  line L1666 (-10075.378, -10016.662) -> (-10075.4372, -10016.4857)
  line L1667 (-10076.5768, -10016.4857) -> (-10076.5768, -10015.8383)
  line L1668 (-10076.8679, -10015.662) -> (-10076.5768, -10015.8383)
  line L1669 (-10076.5768, -10015.8383) -> (-10075.4372, -10015.8383)
  line L1670 (-10075.378, -10015.662) -> (-10075.4372, -10015.8383)
  line L1671 (-10075.4372, -10015.8383) -> (-10075.4372, -10016.4857)
  ellipse E661 centre (-10076.2961, -10016.162) end of major axis (-10076.2961, -10016.262) minor radius 0.0993
  ellipse E662 centre (-10076.2903, -10016.162) end of major axis (-10076.2903, -10016.262) minor radius 0.0993 (-10076.2903, -10016.262) -> (-10076.2903, -10016.062) ccw
  line L1672 (-10076.2961, -10016.062) -> (-10076.2903, -10016.062)
  line L1673 (-10076.2961, -10016.262) -> (-10076.2903, -10016.262)
  line L1674 (-10076.1295, -10016.012) -> (-10076.4512, -10016.012)
  line L1675 (-10076.1063, -10016.012) -> (-10076.1295, -10016.012)
  line L1676 (-10076.4512, -10016.012) -> (-10076.4512, -10016.312)
  line L1677 (-10076.4512, -10016.312) -> (-10076.1295, -10016.312)
  line L1678 (-10076.1063, -10016.312) -> (-10076.1295, -10016.312)
  line L1679 (-10076.1295, -10016.312) -> (-10076.1295, -10016.012)
  line L1680 (-10076.1063, -10016.312) -> (-10076.1063, -10016.012)
  line L1681 (-10076.0035, -10010.6243) -> (-10076.0036, -10010.6245)
  line L1682 (-10076.0036, -10010.6245) -> (-10075.8049, -10010.6013)
  line L1683 (-10075.8049, -10010.6013) -> (-10075.8339, -10010.353)
  line L1684 (-10075.8339, -10010.353) -> (-10075.8339, -10010.3528)
  line L1685 (-10073.9467, -10010.1323) -> (-10075.8339, -10010.3528)
  line L1686 (-10073.7158, -10010.3851) -> (-10073.719, -10010.3574)
  line L1687 (-10076.0036, -10010.6245) -> (-10075.9732, -10010.8844)
  line L1688 (-10075.5265, -10011.8272) -> (-10073.7727, -10011.6223)
  line L1689 (-10073.6031, -10011.3508) -> (-10073.7191, -10010.3576)
  line L1690 (-10073.9468, -10010.1325) -> (-10075.8339, -10010.353)
  line L1691 (-10073.921, -10010.3528) -> (-10073.9467, -10010.1323)
  line L1692 (-10073.719, -10010.3574) -> (-10073.8157, -10010.3687)
  line L1693 (-10073.9178, -10010.3808) -> (-10073.7191, -10010.3576)
  line L1694 (-10073.9468, -10010.1325) -> (-10073.9178, -10010.3808)
  line L1695 (-10073.9178, -10010.3808) -> (-10073.9177, -10010.3806)
  line L1696 (-10073.7191, -10010.3576) -> (-10073.719, -10010.3574)
  line L1697 (-10073.9467, -10010.1323) -> (-10073.9468, -10010.1325)
  line L1698 (-10073.7727, -10011.6223) -> (-10073.7726, -10011.6222)
  line L1699 (-10073.8017, -10011.374) -> (-10073.7727, -10011.6223)
  line L1700 (-10073.6031, -10011.3508) -> (-10073.8017, -10011.374)
  line L1701 (-10073.603, -10011.3507) -> (-10073.6031, -10011.3508)
  line L1702 (-10075.4902, -10011.5713) -> (-10074.0004, -10011.3972)
  line L1703 (-10075.6063, -10010.5781) -> (-10075.4902, -10011.5713)
  line L1704 (-10074.1164, -10010.404) -> (-10075.6063, -10010.5781)
  line L1705 (-10074.0004, -10011.3972) -> (-10074.1164, -10010.404)
  line L1706 (-10074.1959, -10011.2425) -> (-10075.3355, -10011.3756)
  line L1707 (-10075.4902, -10011.5713) -> (-10075.3355, -10011.3756)
  line L1708 (-10074.0004, -10011.3972) -> (-10074.1959, -10011.2425)
  line L1709 (-10075.3355, -10011.3756) -> (-10075.4106, -10010.7326)
  line L1710 (-10075.6063, -10010.5781) -> (-10075.4106, -10010.7326)
  line L1711 (-10075.4106, -10010.7326) -> (-10074.271, -10010.5995)
  line L1712 (-10074.1164, -10010.404) -> (-10074.271, -10010.5995)
  line L1713 (-10074.271, -10010.5995) -> (-10074.1959, -10011.2425)
  circle A35 centre (-10075.0634, -10011.018) radius 0.1
  line L1714 (-10074.92, -10010.8502) -> (-10075.2416, -10010.8878)
  line L1715 (-10074.92, -10010.8502) -> (-10074.92, -10010.8502)
  line L1716 (-10074.92, -10010.8502) -> (-10075.2416, -10010.8877)
  line L1717 (-10075.2416, -10010.8877) -> (-10075.2416, -10010.8878)
  line L1718 (-10075.2416, -10010.8878) -> (-10075.2068, -10011.1857)
  line L1719 (-10075.2068, -10011.1857) -> (-10074.8852, -10011.1482)
  line L1720 (-10074.8852, -10011.1481) -> (-10074.8852, -10011.1482)
  line L1721 (-10074.8852, -10011.1482) -> (-10074.92, -10010.8502)
  line L1722 (-10074.8852, -10011.1481) -> (-10074.92, -10010.8502)
  line L1723 (-10080.8297, -10015.662) -> (-10080.6306, -10015.662)
  line L1724 (-10080.6306, -10015.662) -> (-10080.6306, -10015.412)
  line L1725 (-10080.6306, -10016.662) -> (-10080.8297, -10016.662)
  line L1726 (-10080.6306, -10016.912) -> (-10080.6306, -10016.662)
  line L1727 (-10080.8297, -10015.662) -> (-10080.8297, -10016.662)
  line L1728 (-10080.6306, -10016.912) -> (-10078.8245, -10016.912)
  line L1729 (-10078.8245, -10015.412) -> (-10080.6306, -10015.412)
  line L1730 (-10080.4314, -10016.662) -> (-10079.0234, -10016.662)
  line L1731 (-10080.4314, -10015.662) -> (-10080.4314, -10016.662)
  line L1732 (-10079.0234, -10015.662) -> (-10080.4314, -10015.662)
  line L1733 (-10079.6809, -10016.4857) -> (-10080.1616, -10016.4857)
  line L1734 (-10080.4314, -10016.662) -> (-10080.1616, -10016.4857)
  line L1735 (-10080.1616, -10016.4857) -> (-10080.1616, -10015.8383)
  line L1736 (-10080.4314, -10015.662) -> (-10080.1616, -10015.8383)
  line L1737 (-10080.1616, -10015.8383) -> (-10079.6809, -10015.8383)
  ellipse E663 centre (-10079.8748, -10016.162) end of major axis (-10079.8748, -10016.262) minor radius 0.0996
  ellipse E664 centre (-10079.8701, -10016.162) end of major axis (-10079.8701, -10016.262) minor radius 0.0996 (-10079.8701, -10016.262) -> (-10079.8701, -10016.062) ccw
  line L1738 (-10079.8748, -10016.062) -> (-10079.8701, -10016.062)
  line L1739 (-10079.8748, -10016.262) -> (-10079.8701, -10016.262)
  line L1740 (-10079.7089, -10016.012) -> (-10080.0313, -10016.012)
  line L1741 (-10079.69, -10016.012) -> (-10079.7089, -10016.012)
  line L1742 (-10080.0313, -10016.012) -> (-10080.0313, -10016.312)
  line L1743 (-10080.0313, -10016.312) -> (-10079.7089, -10016.312)
  line L1744 (-10079.69, -10016.312) -> (-10079.7089, -10016.312)
  line L1745 (-10079.7089, -10016.312) -> (-10079.7089, -10016.012)
  line L1746 (-10079.69, -10016.312) -> (-10079.69, -10016.012)
  line L1747 (-10079.6036, -10011.9003) -> (-10079.8027, -10011.9192)
  line L1748 (-10079.8027, -10011.9192) -> (-10079.8027, -10011.9193)
  line L1749 (-10079.8027, -10011.9193) -> (-10079.6036, -10011.9004)
  line L1750 (-10079.6036, -10011.9004) -> (-10079.6272, -10011.6515)
  line L1751 (-10079.6272, -10011.6515) -> (-10079.6272, -10011.6514)
  line L1752 (-10079.5092, -10012.8959) -> (-10079.7083, -10012.9148)
  line L1753 (-10079.4856, -10013.1448) -> (-10079.5092, -10012.8959)
  line L1754 (-10079.407, -10011.6306) -> (-10079.6272, -10011.6514)
  line L1755 (-10079.8027, -10011.9193) -> (-10079.7083, -10012.9148)
  line L1756 (-10079.4856, -10013.1448) -> (-10077.5941, -10012.9655)
  line L1757 (-10077.4186, -10012.6978) -> (-10077.433, -10012.5453)
  line L1758 (-10077.8748, -10011.4854) -> (-10079.6272, -10011.6515)
  line L1759 (-10077.5941, -10012.9655) -> (-10077.5941, -10012.9654)
  line L1760 (-10077.6177, -10012.7167) -> (-10077.5941, -10012.9655)
  line L1761 (-10077.4186, -10012.6978) -> (-10077.6177, -10012.7167)
  line L1762 (-10077.4186, -10012.6977) -> (-10077.4186, -10012.6978)
  line L1763 (-10079.3101, -10012.8771) -> (-10077.8168, -10012.7355)
  line L1764 (-10079.4045, -10011.8815) -> (-10079.3101, -10012.8771)
  line L1765 (-10077.9112, -10011.74) -> (-10079.4045, -10011.8815)
  line L1766 (-10077.8168, -10012.7355) -> (-10077.9112, -10011.74)
  line L1767 (-10078.009, -10012.5765) -> (-10079.1512, -10012.6848)
  line L1768 (-10079.3101, -10012.8771) -> (-10079.1512, -10012.6848)
  line L1769 (-10077.8168, -10012.7355) -> (-10078.009, -10012.5765)
  line L1770 (-10079.1512, -10012.6848) -> (-10079.2123, -10012.0404)
  line L1771 (-10079.4045, -10011.8815) -> (-10079.2123, -10012.0404)
  line L1772 (-10079.2123, -10012.0404) -> (-10078.0701, -10011.9321)
  line L1773 (-10077.9112, -10011.74) -> (-10078.0701, -10011.9321)
  line L1774 (-10078.0701, -10011.9321) -> (-10078.009, -10012.5765)
  circle A36 centre (-10078.8714, -10012.3332) radius 0.1
  line L1775 (-10078.7243, -10012.1686) -> (-10079.0467, -10012.1991)
  line L1776 (-10078.7243, -10012.1686) -> (-10079.0467, -10012.1991)
  line L1777 (-10079.0467, -10012.1991) -> (-10079.0184, -10012.4978)
  line L1778 (-10079.0184, -10012.4978) -> (-10078.696, -10012.4672)
  line L1779 (-10078.696, -10012.4672) -> (-10078.7243, -10012.1686)
  ellipse E665 centre (-10075.7301, -10029.6225) end of major axis (-10075.6695, -10030.8209) minor radius 0.2145 (-10075.9337, -10028.8658) -> (-10075.6316, -10030.799) ccw
  ellipse E666 centre (-10075.5336, -10029.6125) end of major axis (-10075.4831, -10030.6112) minor radius 0.1787 (-10075.7111, -10029.0805) -> (-10075.3848, -10030.3988) ccw
  line L1780 (-10075.4515, -10030.593) -> (-10075.6316, -10030.799)
  ellipse E667 centre (-10075.5336, -10029.6125) end of major axis (-10075.4957, -10030.3616) minor radius 0.134 (-10075.6719, -10029.3371) -> (-10075.4141, -10030.152) ccw
  line L1781 (-10075.6695, -10030.8209) -> (-10076.518, -10030.8638)
  ellipse E668 centre (-10075.7301, -10008.5715) end of major axis (-10075.6695, -10007.3731) minor radius 0.2145 (-10075.6316, -10007.395) -> (-10075.9337, -10009.3282) ccw
  ellipse E669 centre (-10075.5336, -10008.5815) end of major axis (-10075.4831, -10007.5827) minor radius 0.1787 (-10075.3848, -10007.7952) -> (-10075.7111, -10009.1135) ccw
  line L1782 (-10075.4515, -10007.601) -> (-10075.6316, -10007.395)
  ellipse E670 centre (-10075.5336, -10008.5815) end of major axis (-10075.4957, -10007.8324) minor radius 0.134 (-10075.4141, -10008.042) -> (-10075.6719, -10008.8569) ccw
  line L1783 (-10075.6695, -10007.3731) -> (-10076.518, -10007.3302)
  ellipse E671 centre (-10090.4171, -10019.097) end of major axis (-10090.4171, -10019.6634) minor radius 0.5639 (-10089.9892, -10018.728) -> (-10089.9892, -10019.466) ccw
  line L1784 (-10090.8099, -10019.2106) -> (-10090.7114, -10018.8121)
  line L1785 (-10090.7114, -10018.8121) -> (-10090.3186, -10018.6985)
  line L1786 (-10090.3186, -10018.6985) -> (-10090.0482, -10018.9602)
  line L1787 (-10090.0807, -10019.2118) -> (-10090.1227, -10019.3819)
  line L1788 (-10090.1227, -10019.3819) -> (-10090.5155, -10019.4955)
  line L1789 (-10090.5155, -10019.4955) -> (-10090.8099, -10019.2106)
  line L1790 (-10090.7114, -10018.8121) -> (-10090.6217, -10018.8121)
  line L1791 (-10090.7206, -10019.2106) -> (-10090.8099, -10019.2106)
  spline S53 degree 3 poles (-10045.5969, -10030.692) (-10045.5963, -10030.6873) (-10045.5949, -10030.677) (-10045.5853, -10030.6623) (-10045.5707, -10030.6477) (-10045.5504, -10030.6334) (-10045.5248, -10030.6195) (-10045.482, -10030.6008) (-10045.433, -10030.585) (-10045.3785, -10030.5714) (-10045.3141, -10030.5581) (-10045.2258, -10030.5447) (-10045.1146, -10030.5354) (-10045, -10030.532) (-10044.8854, -10030.5354) (-10044.7742, -10030.5447) (-10044.6859, -10030.5581) (-10044.6215, -10030.5714) (-10044.567, -10030.585) (-10044.518, -10030.6008) (-10044.4752, -10030.6195) (-10044.4496, -10030.6334) (-10044.4293, -10030.6477) (-10044.4147, -10030.6623) (-10044.4051, -10030.677) (-10044.4037, -10030.6873) (-10044.4031, -10030.692) knots 0 0 0 0 0.011067 0.024078 0.039928 0.05914 0.081934 0.10802 0.168059 0.202015 0.239296 0.321668 0.410563 0.5 0.589437 0.678332 0.760704 0.797985 0.831941 0.89198 0.918066 0.94086 0.960072 0.975922 0.988933 1 1 1 1